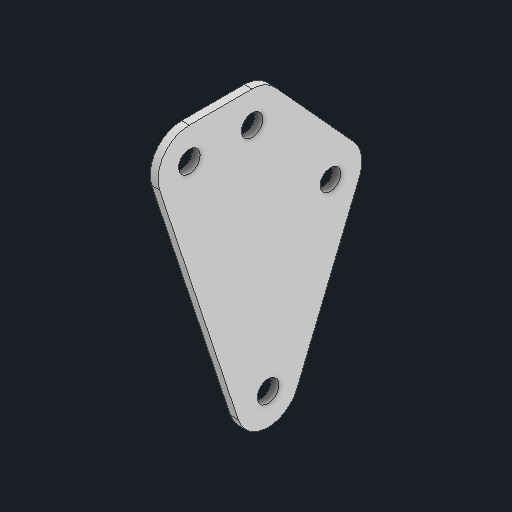
# Autodesk Inventor part: bottom_joint_gusset
Saved by Autodesk Inventor 2025 (Build 290162000, 162)
## iProperties
Created: 2024-10-13
Part Number: bottom_joint_gusset
Material: Generic
Document SubType Name: Modeling
Designer: Averey Ku
Density: 1 g/cm^3
Appearance: Default
Author: Averey Ku
Autodesk Inventor part; units mm, degrees
ref_plane "YZ Plane" through (0, 0, 0) normal (1, 0, 0) x (0, 1, 0)
ref_plane "XZ Plane" through (0, 0, 0) normal (0, 1, 0) x (-1, 0, 0)
ref_plane "XY Plane" through (0, 0, 0) normal (0, 0, 1) x (1, 0, 0)
sketch "maiin" plane through (0, 0, 0) normal (0, 0, 1) x (1, 0, 0)
  circle A0 centre (-0.0182, -20.0228) radius 2.1844
  circle A1 centre (12.6818, -20.0228) radius 2.1844
  circle A2 centre (-3.2386, 28.228) radius 2.1844 construction
  arc A3 (-4.7148, -24.2902) -> (-0.0224, -26.3686) centre (-0.0182, -20.0228) ccw
  arc A4 (12.6776, -26.377) -> (18.7159, -18.0313) centre (12.6818, -20.0228) ccw
  arc A5 (2.7914, 30.2182) -> (-9.112, 30.6417) centre (-3.2386, 28.228) ccw
  arc A6 (-21.7607, -0.1371) -> (-20.5872, -6.821) centre (-15.8874, -2.5508) ccw
  circle A7 centre (-15.8874, -2.5508) radius 2.0955
  line L0 (18.7159, -18.0313) -> (2.7914, 30.2182)
  line L1 (12.6776, -26.377) -> (-0.0224, -26.3686)
  line L2 (-4.7148, -24.2902) -> (-20.5872, -6.821)
  line L3 (-9.112, 30.6417) -> (-21.7607, -0.1371)
  circle A8 centre (-3.2386, 28.228) radius 2.1844
  point P0 (3.1417, -3.9392)
  dimension "d0" = 12.7
  dimension "d1" = 12.7
  dimension "d2" = 4.191
  dimension "d3" = 4.3688
  measures "d0" diameter of A5
  measures "d1" diameter of A6
  measures "d2" diameter of A7
  measures "d3" diameter of A8
sketch "Sketch1" plane through (0, 0, 0) normal (1, 0, 0) x (0, 1, 0)
  circle A0 centre (0.0042, -12.7) radius 2.1844
  circle A1 centre (0, 0) radius 2.1844
  circle A2 centre (-48.2455, -15.9365) radius 2.1844 construction
  arc A3 (4.2731, -17.3952) -> (6.35, -12.7021) centre (0.0042, -12.7) ccw
  arc A4 (6.3542, -0.0021) -> (-1.9935, 6.0334) centre (0, 0) ccw
  arc A5 (-50.2377, -9.9071) -> (-50.6573, -21.8107) centre (-48.2455, -15.9365) ccw
  arc A6 (-19.8742, -34.4492) -> (-13.1908, -33.2734) centre (-17.4625, -28.575) ccw
  circle A7 centre (-17.4625, -28.575) radius 2.0955
  line L0 (-1.9935, 6.0334) -> (-50.2377, -9.9071)
  line L1 (6.3542, -0.0021) -> (6.35, -12.7021)
  line L2 (4.2731, -17.3952) -> (-13.1908, -33.2734)
  line L3 (-50.6573, -21.8107) -> (-19.8742, -34.4492)
  circle A8 centre (-48.2455, -15.9365) radius 2.1844
  point P0 (0, 0)
  constraints: 1 other
extrude "Extrusion1" add sketch "Sketch1" along normal blind 1.5875
body "Solid1"
